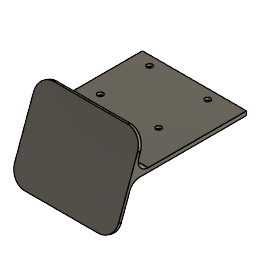
Pi Cover Top (Autodesk Fusion 360 design; units mm, degrees)
Autodesk Fusion 360 part; units mm, degrees
sketch "Sketch1" plane through (0, 0, 0) normal (0, 0, 1) x (1, 0, 0)
  line L0 (-51.9, 32.75) -> (51.9, 32.75)
  line L1 (51.9, 32.75) -> (51.9, -32.75)
  line L2 (51.9, -32.75) -> (-51.9, -32.75)
  line L3 (-51.9, -32.75) -> (-51.9, 32.75)
  point P0 (0, 32.75)
  point P1 (51.9, 0)
  dimension "d1" = 103.8
  dimension "d2" = 65.5
  constraint horizontal L0
  constraint vertical L1
  constraint horizontal L2
  constraint vertical L3
  constraint midpoint L0 P0
  constraint midpoint L1 P1
  constraint vertical origin P0
  constraint horizontal origin P1
  measures "d1" distance of L0.start L0.end
  measures "d2" distance of L0.end L1.end
extrude "Extrude1" add sketch "Sketch1" along normal mid plane 4
sketch "Sketch2" plane through (0, 0, 2) normal (0, 0, 1) x (-1, 0, 0)
  line L0 (51.9, 32.75) -> (-51.9, 32.75)
  line L1 (-51.9, 32.75) -> (-51.9, -32.75)
  line L2 (-51.9, -32.75) -> (51.9, -32.75)
  line L3 (51.9, -32.75) -> (51.9, 32.75)
  point P0 (35.3, -23.25)
  point P1 (-22.7, -23.25)
  point P2 (35.3, 25.75)
  point P3 (-22.7, 25.75)
  dimension "d5" = 9.5
  dimension "d6" = 16.6
  dimension "d7" = 58
  dimension "d8" = 49
  constraint horizontal P0 P1
  constraint vertical P0 P2
  constraint vertical P1 P3
  constraint horizontal P2 P3
  measures "d5" distance of L2 P0
  measures "d6" distance of L3 P0
  measures "d7" horizontal distance of P0 P1
  measures "d8" vertical distance of P0 P2
hole "Hole1" at (-35.3, 23.25, 2) at (22.7, 23.25, 2) at (22.7, -25.75, 2) at (-35.3, -25.75, 2) direction (0, 0, -1) diameter 2.9 depth 12 tip angle 118 counterbore diameter 5.5 counterbore depth 2.5
sketch "Sketch3" plane through (0, 0, -2) normal (0, 0, -1) x (1, 0, 0)
  circle A0 centre (22.7, 25.75) radius 1.45
  circle A1 centre (-35.3, -23.25) radius 1.45
  circle A2 centre (22.7, -23.25) radius 1.45
  circle A3 centre (-35.3, 25.75) radius 1.45
  line L0 (51.9, 32.75) -> (-51.9, 32.75)
  line L1 (-51.9, 32.75) -> (-51.9, -32.75)
  line L2 (-51.9, -32.75) -> (51.9, -32.75)
  line L3 (51.9, -32.75) -> (51.9, 32.75)
  line L4 (-48.775, 31.125) -> (50.275, 31.125)
  line L5 (50.275, 31.125) -> (50.275, -29.625)
  line L6 (50.275, -29.625) -> (-48.775, -29.625)
  line L7 (-48.775, -29.625) -> (-48.775, 31.125)
  line L8 (-46.775, 29.125) -> (48.275, 29.125)
  line L9 (48.275, 29.125) -> (48.275, -27.625)
  line L10 (48.275, -27.625) -> (-46.775, -27.625)
  line L11 (-46.775, -27.625) -> (-46.775, 29.125)
  point P0 (0.75, 31.125)
  point P1 (0.75, 29.125)
  point P2 (50.275, 0.75)
  point P3 (48.275, 0.75)
  dimension "d14" = 2
  dimension "d15" = 2
  dimension "d16" = 99.05
  dimension "d17" = 60.75
  dimension "d41" = 3.125
  dimension "d42" = 1.625
  constraint horizontal L4
  constraint vertical L5
  constraint horizontal L6
  constraint vertical L7
  constraint horizontal L8
  constraint vertical L9
  constraint horizontal L10
  constraint vertical L11
  constraint midpoint L4 P0
  constraint midpoint L8 P1
  constraint midpoint L5 P2
  constraint midpoint L9 P3
  constraint vertical P0 P1
  constraint horizontal P2 P3
  measures "d14" distance of L4 L8
  measures "d15" distance of L7 L11
  measures "d16" distance of L4.start L4.end
  measures "d17" distance of L4.start L6.end
  measures "d41" distance of L1 L7
  measures "d42" distance of L0 L4
extrude "Extrude2" add sketch "Sketch3" along normal blind 1 contours L4 L5 L6 L7
sketch "Sketch5" plane through (0, 0, 2) normal (0, 0, 1) x (-1, 0, 0)
  circle A0 centre (-22.7, 25.75) radius 2.75
  circle A1 centre (35.3, -23.25) radius 2.75
  circle A2 centre (-22.7, -23.25) radius 2.75
  circle A3 centre (35.3, 25.75) radius 2.75
  line L0 (51.9, 32.75) -> (-51.9, 32.75)
  line L1 (-51.9, 32.75) -> (-51.9, -32.75)
  line L2 (-51.9, -32.75) -> (51.9, -32.75)
  line L3 (51.9, -32.75) -> (51.9, 32.75)
  line L4 (51.9, 32.75) -> (-51.9, 32.75)
  line L5 (-51.9, 32.75) -> (-51.9, 82.75)
  line L6 (-51.9, 82.75) -> (51.9, 82.75)
  line L7 (51.9, 82.75) -> (51.9, 32.75)
  dimension "d20" = 50
  constraint horizontal L4
  constraint vertical L5
  constraint horizontal L6
  constraint vertical L7
  constraint coincident L0.start L3.end
  constraint coincident L0.end L5
  measures "d20" distance of L0.end L5.end
extrude "Extrude3" add sketch "Sketch5" against normal up to surface (4 mm away) contours L0 L4 L5 L6 L7
sketch "Sketch7" plane through (-51.9, 0, 0) normal (-1, 0, 0) x (0, -1, 0)
  line L0 (82.75, 2) -> (-32.75, 2)
  line L1 (-32.75, 2) -> (-32.75, -2)
  line L2 (-32.75, -2) -> (82.75, -2)
  line L3 (82.75, -2) -> (82.75, 2)
  line L4 (82.75, 2) -> (99.851, -44.9846)
  line L5 (99.851, -44.9846) -> (97.0319, -46.0107)
  line L6 (97.0319, -46.0107) -> (81.0133, -2)
  line L7 (82.75, 2) -> (70.7793, 34.8892)
  line L8 (70.7793, 34.8892) -> (67.9602, 33.8632)
  line L9 (67.9602, 33.8632) -> (81.0133, -2)
  dimension "d23" = 70
  dimension "d24" = 50
  dimension "d27" = 3
  dimension "d28" = 35
  constraint coincident L0.start L3.end
  constraint perpendicular L4 L5
  constraint parallel L4 L6
  constraint coincident L2 L6.end
  constraint perpendicular L7 L8
  constraint parallel L7 L9
  constraint coincident L4 L7.end
  measures "d23" angle of L0 L4
  measures "d24" distance of L0.start L4.end
  measures "d27" distance of L4.end L5.end
  measures "d28" distance of L0.start L7.end
extrude "Extrude4" add sketch "Sketch7" against normal up to surface (103.8 mm away) contours L2 L3 L4 L5 L6 | L0 L7 L8 L9
fillet "Fillet1" radius 15 4 edges at (-51.9, -69.3698, 34.3762) (51.9, -69.3698, 34.3762) (51.9, -98.4415, -45.4977) (-51.9, -98.4415, -45.4977)
fillet "Fillet2" radius 10 2 edges at (0, -81.0133, -2) (0, -79.5575, 2)
sketch "Sketch8" plane through (0, 0, 2) normal (0, 0, 1) x (-1, 0, 0)
  line L0 (51.9, 65.276) -> (-51.9, 65.276)
  line L1 (-51.9, 65.276) -> (-51.9, -32.75)
  line L2 (-51.9, -32.75) -> (51.9, -32.75)
  line L3 (51.9, -32.75) -> (51.9, 65.276)
  circle A0 centre (-22.7, 25.75) radius 2.75
  circle A1 centre (35.3, -23.25) radius 2.75
  circle A2 centre (-22.7, -23.25) radius 2.75
  circle A3 centre (35.3, 25.75) radius 2.75
  line L4 (15, 49.276) -> (-15, 49.276)
  line L5 (-15, 49.276) -> (-15, 64.276)
  line L6 (-15, 64.276) -> (15, 64.276)
  line L7 (15, 64.276) -> (15, 49.276)
  point P0 (0, 49.276)
  dimension "d33" = 1
  dimension "d34" = 15
  dimension "d35" = 30
  constraint horizontal L4
  constraint vertical L5
  constraint horizontal L6
  constraint vertical L7
  constraint midpoint L4 P0
  constraint vertical origin P0
  measures "d33" distance of L0 L6
  measures "d34" distance of L4.end L5.end
  measures "d35" distance of L4.start L4.end
extrude "Extrude5" cut sketch "Sketch8" against normal up to surface (4 mm away) contours L4 L5 L6 L7
fillet "Fillet3" radius 5 4 edges at (-15, -64.276, 0) (15, -64.276, 0) (15, -49.276, 0) (-15, -49.276, 0)
equation "d15 = d14"
equation "d16 = 99.30 mm - 0.25 mm"
equation "d17 = 61.00 mm - 0.25 mm"
equation "d41 = 3 mm + ( 0.25 / 2 ) * 1 mm"
equation "d42 = 1.5 mm + ( 0.25 / 2 ) * 1 mm"
